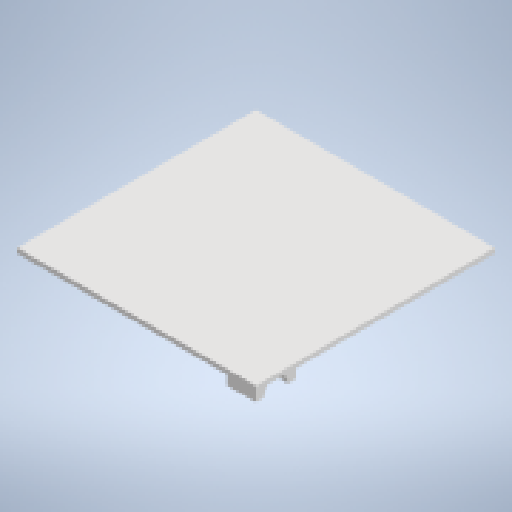
# Autodesk Inventor part: plateauV2102
Saved by Autodesk Inventor 2025.2 (Build 292293000, 293)
## iProperties
Created: 2025-02-21
Part Number: plateauV2102
Material: Générique
Document SubType Name: Modeling
Designer: antoi
Density: 1 g/cm^3
Appearance: Par défaut
Author: antoi
Autodesk Inventor part; units mm, degrees
ref_plane "YZ Plane" through (0, 0, 0) normal (1, 0, 0) x (0, 1, 0)
ref_plane "XZ Plane" through (0, 0, 0) normal (0, 1, 0) x (-1, 0, 0)
ref_plane "XY Plane" through (0, 0, 0) normal (0, 0, 1) x (1, 0, 0)
sketch "Esquisse1" plane through (0, 0, 0) normal (0, 1, 0) x (-1, 0, 0)
  line L0 (0, 0) -> (150, 0)
  line L1 (150, 0) -> (150, -150)
  line L2 (150, -150) -> (0, -150)
  line L3 (0, -150) -> (0, 0)
  dimension "d0" = 150
  dimension "d1" = 150
  constraints: 8 end point, 2 parallel, 1 horizontal, 1 perpendicular
  measures "d0" distance of L1.end L2.end
  measures "d1" distance of L0.end L1.end
extrude "Extrusion1" add sketch "Esquisse1" along normal blind 3
sketch "Esquisse2" plane through (0, 0, 0) normal (1, 0, 0) x (0, 0, -1)
  line L0 (0, 0) -> (35, 0)
  line L1 (35, 0) -> (35, -5.9)
  line L2 (0, -5.9) -> (0, 0)
  arc A0 (25.2, -5.9) -> (22.4477, 0) centre (17.5, -5.9) ccw
  arc A1 (12.5523, 0) -> (9.8, -5.9) centre (17.5, -5.9) ccw
  line L3 (35, -5.9) -> (25.2, -5.9)
  line L4 (9.8, -5.9) -> (0, -5.9)
  point P0 (17.4477, 0)
  point P1 (7.5523, 0)
  point P2 (5.9342, -5.9)
  point P3 (23.4002, -5.9)
  dimension "d4" = 35
  dimension "d5" = 5.9
  constraints: 10 end point, 5 point on line, 4 point on circle, 3 parallel, 2 centre point, 1 horizontal, 1 perpendicular
  measures "d4" distance of L1.end L2.start
  measures "d5" distance of L0.end L1.end
extrude "Extrusion2" add sketch "Esquisse2" against normal blind 18.6
ref_plane "Plan de construction1" through (-150, 3, -4.9) normal (0, 0, 1) x (1, 0, 0)
ref_plane "Plan de construction2" through (0, -5.9, -30.1) normal (0, 0, -1) x (-1, 0, 0)
ref_plane "Plan de construction3" through (-4.5, 3, 0) normal (1, 0, 0) x (0, 0, -1)
ref_plane "Plan de construction4" through (-14.1, 3, 0) normal (1, 0, 0) x (0, 0, -1)
hole "Perçage1" at (-14.1, -5.9, -30.1) direction (0, 1, 0) diameter 6.3 depth 8.1
hole "Perçage2" at (-4.5, -5.9, -30.1) direction (0, 1, 0) diameter 6.3 depth 8.1
hole "Perçage3" at (-4.5, -5.9, -4.9) direction (0, 1, 0) diameter 6.3 depth 8.1
hole "Perçage4" at (-14.1, -5.9, -4.9) direction (0, 1, 0) diameter 6.3 depth 8.1
pattern_linear "Réseau rectangulaire1" count 2 spacing 115 along (0, 0, -1) count 2 spacing 131.4 along (-1, 0, 0) of "Extrusion2", "Perçage2", "Perçage1", "Perçage3", "Perçage4"
